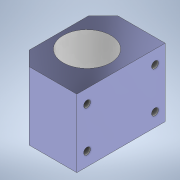
# Autodesk Inventor part: Soporte Tuerca
Saved by Autodesk Inventor 2021 (Build 250183000, 183)
## iProperties
Created: 2022-01-21
Part Number: Soporte Tuerca
Material: Generic
Document SubType Name: Modeling
Designer: deuts
Density: 1 g/cm^3
Appearance: Default
Author: deuts
Autodesk Inventor part; units mm, degrees
ref_plane "YZ Plane" through (0, 0, 0) normal (1, 0, 0) x (0, 1, 0)
ref_plane "XZ Plane" through (0, 0, 0) normal (0, 1, 0) x (-1, 0, 0)
ref_plane "XY Plane" through (0, 0, 0) normal (0, 0, 1) x (1, 0, 0)
sketch "Sketch1" plane through (0, 0, 0) normal (0, 1, 0) x (-1, 0, 0)
  circle A0 centre (0, 0) radius 14
  line L0 (0, 0) -> (-20, 0)
  line L1 (-20, 0) -> (-20, -26)
  line L2 (-20, -26) -> (8, -26)
  line L3 (8, -26) -> (16.4853, -17.5147)
  line L4 (-20, 0) -> (-20, 26)
  line L5 (-20, 26) -> (8, 26)
  line L6 (8, 26) -> (16.4853, 17.5147)
  line L7 (16.4853, 17.5147) -> (16.4853, -17.5147)
  dimension "d0" = 28
  dimension "d1" = 20
  dimension "d2" = 26
  dimension "d3" = 28
  dimension "d4" = 12
  dimension "d5" = 135
  dimension "d6" = 28
  dimension "d7" = 26
  dimension "d8" = 12
  constraints: 16 end point, 3 perpendicular, 1 centre point, 1 coincident, 1 horizontal, 1 vertical
  measures "d0" diameter of A0
  measures "d1" distance of L0.start L0.end
  measures "d2" distance of L0.end L1.end
  measures "d3" distance of L1.end L2.end
  measures "d4" distance of L2.end L3.end
  measures "d5" angle of L3 L2
  measures "d6" distance of L4.end L5.end
  measures "d7" distance of L0.end L4.end
  measures "d8" distance of L5.end L6.end
extrude "Extrusion1" add sketch "Sketch1" along normal blind 40
sketch "Sketch2" plane through (20, 0, 26) normal (1, 0, 0) x (0, 0, -1)
  line L0 (0, 0) -> (0, 40) projected
  line L1 (0, 40) -> (0, 32)
  circle A0 centre (6, 32) radius 2
  point P0 (26, 0)
  dimension "d11" = 8
  dimension "d13" = 4
  constraints: 2 end point, 1 centre point, 1 point on line
  measures "d11" distance of L0.end L1.end
  measures "d13" diameter of A0
extrude "Extrusion2" cut sketch "Sketch2" against normal blind 15
pattern_linear "Rectangular Pattern1" count 2 spacing 24 along (0, -1, 0) count 2 spacing 40 along (0, 0, -1) of "Extrusion2"
body "Solid1"
